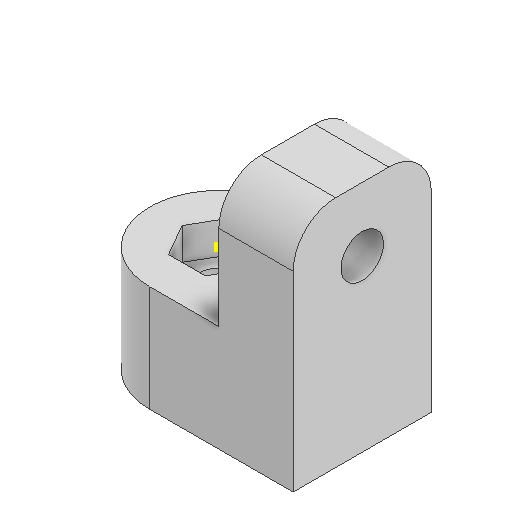
# Autodesk Inventor part: SpringConn
Saved by Autodesk Inventor 2022 (Build 260153000, 153)
## iProperties
Created: 2022-11-22
Part Number: SpringConn
Material: Generic
Document SubType Name: Modeling
Designer: MVeszpremi
Density: 1 g/cm^3
Appearance: Default
Author: MVeszpremi
Autodesk Inventor part; units mm, degrees
ref_plane "XZ Plane" through (0, 0, 0) normal (0, 1, 0) x (-1, 0, 0)
ref_plane "XY Plane" through (0, 0, 0) normal (0, 0, 1) x (1, 0, 0)
sketch "Sketch1" plane through (0, 0, 0) normal (0, 1, 0) x (-1, 0, 0)
  circle A0 centre (0, 0) radius 6.5
  circle A1 centre (0, 0) radius 1.8
  dimension "d0" = 13
  dimension "d1" = 3.6
  constraints: 2 centre point, 2 coincident
  measures "d0" diameter of A0
  measures "d1" diameter of A1
extrude "Extrusion1" add sketch "Sketch1" along normal blind 10
sketch "Sketch2" plane through (0, 10, 0) normal (0, 1, 0) x (1, 0, 0)
  point P0 (0, 0)
ref_plane "Work Plane1" through (6.5, 0, 0) normal (1, 0, 0) x (0, 1, 0)
sketch "Sketch3" plane through (6.5, 0, 0) normal (1, 0, 0) x (0, 1, 0)
  line L0 (10, -6.5) -> (10, 6.5) projected
  line L1 (10, -6.5) -> (22, -6.5)
  line L2 (22, -6.5) -> (22, 6.5)
  line L3 (22, 6.5) -> (10, 6.5)
  line L4 (10, 6.5) -> (10, -6.5)
  line L5 (0, -6.5) -> (0, 6.5) projected
  line L6 (10, -6.5) -> (0, -6.5)
  line L7 (0, -6.5) -> (0, 6.5)
  line L8 (0, 6.5) -> (10, 6.5)
  line L9 (10, 6.5) -> (10, -6.5)
  circle A0 centre (16, 0) radius 2
  point P0 (0, 0)
  point P1 (0, -6.5)
  point P2 (10, 6.5)
  point P3 (10, 6.5)
  dimension "d5" = 12
  dimension "d6" = 4
  dimension "d11" = 6
  constraints: 16 end point, 4 parallel, 2 horizontal, 2 perpendicular, 1 centre point
  measures "d5" distance of L0.start L1.end
  measures "d6" diameter of A0
  measures "d11" distance from line of L0 A0.centre
extrude "Extrusion2" add sketch "Sketch3" against normal up to surface contours L6 L5 L8 L0 round surface about axis through (0, 0, 0) along (0, 1, 0) radius 6.5 far side no
extrude "Extrusion3" add sketch "Sketch3" along normal blind 7
sketch "Sketch5" plane through (0, 10, 0) normal (0, 1, 0) x (1, 0, 0)
  line L0 (3.4641, 0) -> (1.7321, -3)
  line L1 (1.7321, -3) -> (-1.7321, -3)
  line L2 (-1.7321, -3) -> (-3.4641, 0)
  line L3 (-3.4641, 0) -> (-1.7321, 3)
  line L4 (-1.7321, 3) -> (1.7321, 3)
  line L5 (1.7321, 3) -> (3.4641, 0)
  point P0 (0, 0)
  point P1 (0, 0)
  dimension "d12" = 6
  constraints: 12 end point, 1 coincident, 13 other
  measures "d12" distance between parallel lines of L4 L1
extrude "Extrusion4" cut sketch "Sketch5" against normal blind 3
fillet "Fillet1" radius 4 2 edges at (10, 22, 6.5) (10, 22, -6.5)
sketch "Sketch6" plane through (6.5, 0, 0) normal (-1, 0, 0) x (0, 0, 1)
  circle A0 centre (0, 16) radius 2 projected
  circle A1 centre (0, 16) radius 4
  point P0 (0, 0)
  dimension "d16" = 8
  constraints: 1 centre point, 1 coincident
  measures "d16" diameter of A1
extrude "Extrusion5" cut sketch "Sketch6" against normal blind 2
body "Solid1"
